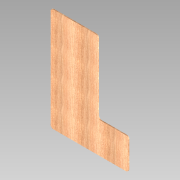
# Autodesk Inventor part: 4102_Mounting Plate_V1
Saved by Autodesk Inventor 2020 (Build 240168000, 168)
## iProperties
Created: 2020-09-10
Part Number: 4102_Mounting Plate_V1
Material: Wood (Birch)
Document SubType Name: Modeling
Designer: Eli Mattingly
Density: 0.55 g/cm^3
Appearance: Birch - Natural Polished
Author: Eli Mattingly
Autodesk Inventor part; units mm, degrees
ref_plane "YZ Plane" through (0, 0, 0) normal (1, 0, 0) x (0, 1, 0)
ref_plane "XZ Plane" through (0, 0, 0) normal (0, 1, 0) x (-1, 0, 0)
ref_plane "XY Plane" through (0, 0, 0) normal (0, 0, 1) x (1, 0, 0)
sketch "Sketch1" plane through (0, 0, 0) normal (0, 0, 1) x (1, 0, 0)
  line L0 (-375, 500) -> (375, 500)
  line L1 (375, 500) -> (375, -500)
  line L2 (375, -500) -> (-375, -500)
  line L3 (-375, -500) -> (-375, 500)
  line L4 (-375, 500) -> (375, -500) construction
  line L5 (375, 500) -> (-375, -500) construction
  line L6 (375, 500) -> (82.2, 500)
  line L7 (82.2, 500) -> (82.2, -200)
  line L8 (82.2, -200) -> (375, -200)
  line L9 (375, -200) -> (375, 500)
  point P0 (0, 0)
  dimension "d0" = 750
  dimension "d1" = 1000
  dimension "d2" = 457.2
  dimension "d3" = 300
  constraints: 20 end point, 4 parallel, 2 horizontal, 2 midpoint, 2 perpendicular
  measures "d0" distance of L1.end L2.end
  measures "d1" distance of L0.end L1.end
  measures "d2" distance between parallel lines of L3 L7
  measures "d3" distance between parallel lines of L2 L8
extrude "Extrusion1" add sketch "Sketch1" along normal blind 10 contours L0 L7 L8 L1 L2 L3
fillet "Fillet1" radius 25 6 edges at (82.2, -200, 5) (375, -200, 5) (375, -500, 5) (-375, -500, 5) (-375, 500, 5) (82.2, 500, 5)
body "Solid1"
